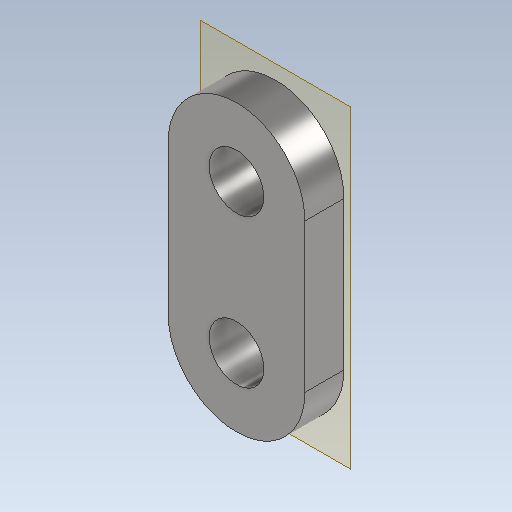
# Autodesk Inventor part: Под стяжку
Saved by Autodesk Inventor 2021 (Build 250183000, 183)
## iProperties
Created: 2020-12-13
Part Number: Под стяжку
Material: Сталь, мягкая
Document SubType Name: Modeling
Designer: Тимоха
Mass: 155.763 g
Surface Area: 67.0768 cm^2
Volume: 19.8424 cm^3
Density: 7.85 g/cm^3
Appearance: С умеренной полировкой
Author: Тимоха
Autodesk Inventor part; units mm, degrees
ref_plane "YZ Plane" through (0, 0, 0) normal (1, 0, 0) x (0, 1, 0)
ref_plane "XZ Plane" through (0, 0, 0) normal (0, 1, 0) x (-1, 0, 0)
ref_plane "XY Plane" through (0, 0, 0) normal (0, 0, 1) x (1, 0, 0)
ref_plane "РабПлоскость1" through (0, 0, 0) normal (0, 0, 1) x (1, 0, 0)
sketch "Эскиз1" plane through (0, 0, 0) normal (0, 0, 1) x (1, 0, 0)
  line L0 (17.5, 19) -> (17.5, -19) projected
  arc A0 (17.5, 19) -> (-17.5, 19) centre (0, 19) ccw projected
  line L1 (-17.5, -19) -> (-17.5, 19) projected
  arc A1 (-17.5, -19) -> (17.5, -19) centre (0, -19) ccw projected
  circle A2 centre (0, -19) radius 7 projected
  circle A3 centre (0, 19) radius 7 projected
  point P0 (0, 0)
extrude "Выдавливание1" add sketch "Эскиз1" along normal blind 10
